Autodesk Fusion 360 part; units mm, degrees
(part 2 of 2)
sketch "20 mm Pickup Opening with Full-Height 45 Degree Bevel Lower Sketch" plane through (0, 0, 2) normal (0, 0, 1) x (1, 0, 0)
  line L0 (111.19, -12) -> (111.19, 37.0643)
  line L1 (111.19, 37.0643) -> (111.2756, 38.3696)
  line L2 (111.2756, 38.3696) -> (111.5307, 39.6525)
  line L3 (111.5307, 39.6525) -> (111.9512, 40.8911)
  line L4 (111.9512, 40.8911) -> (112.5297, 42.0643)
  line L5 (112.5297, 42.0643) -> (113.2565, 43.1519)
  line L6 (113.2565, 43.1519) -> (114.1189, 44.1354)
  line L7 (114.1189, 44.1354) -> (115.1024, 44.9978)
  line L8 (115.1024, 44.9978) -> (116.19, 45.7246)
  line L9 (116.19, 45.7246) -> (117.3632, 46.3031)
  line L10 (117.3632, 46.3031) -> (118.6018, 46.7236)
  line L11 (118.6018, 46.7236) -> (119.8847, 46.9787)
  line L12 (119.8847, 46.9787) -> (121.19, 47.0643)
  line L13 (121.19, 47.0643) -> (122.4953, 46.9787)
  line L14 (122.4953, 46.9787) -> (123.7782, 46.7236)
  line L15 (123.7782, 46.7236) -> (125.0168, 46.3031)
  line L16 (125.0168, 46.3031) -> (126.19, 45.7246)
  line L17 (126.19, 45.7246) -> (127.2776, 44.9978)
  line L18 (127.2776, 44.9978) -> (128.2611, 44.1354)
  line L19 (128.2611, 44.1354) -> (129.1235, 43.1519)
  line L20 (129.1235, 43.1519) -> (129.8503, 42.0643)
  line L21 (129.8503, 42.0643) -> (130.4288, 40.8911)
  line L22 (130.4288, 40.8911) -> (130.8493, 39.6525)
  line L23 (130.8493, 39.6525) -> (131.1044, 38.3696)
  line L24 (131.1044, 38.3696) -> (131.19, 37.0643)
  line L25 (131.19, 37.0643) -> (131.19, -12)
  line L26 (131.19, -12) -> (131.1044, -13.3053)
  line L27 (131.1044, -13.3053) -> (130.8493, -14.5882)
  line L28 (130.8493, -14.5882) -> (130.4288, -15.8268)
  line L29 (130.4288, -15.8268) -> (129.8503, -17)
  line L30 (129.8503, -17) -> (129.1235, -18.0876)
  line L31 (129.1235, -18.0876) -> (128.2611, -19.0711)
  line L32 (128.2611, -19.0711) -> (127.2776, -19.9335)
  line L33 (127.2776, -19.9335) -> (126.19, -20.6603)
  line L34 (126.19, -20.6603) -> (125.0168, -21.2388)
  line L35 (125.0168, -21.2388) -> (123.7782, -21.6593)
  line L36 (123.7782, -21.6593) -> (122.4953, -21.9144)
  line L37 (122.4953, -21.9144) -> (121.19, -22)
  line L38 (121.19, -22) -> (119.8847, -21.9144)
  line L39 (119.8847, -21.9144) -> (118.6018, -21.6593)
  line L40 (118.6018, -21.6593) -> (117.3632, -21.2388)
  line L41 (117.3632, -21.2388) -> (116.19, -20.6603)
  line L42 (116.19, -20.6603) -> (115.1024, -19.9335)
  line L43 (115.1024, -19.9335) -> (114.1189, -19.0711)
  line L44 (114.1189, -19.0711) -> (113.2565, -18.0876)
  line L45 (113.2565, -18.0876) -> (112.5297, -17)
  line L46 (112.5297, -17) -> (111.9512, -15.8268)
  line L47 (111.9512, -15.8268) -> (111.5307, -14.5882)
  line L48 (111.5307, -14.5882) -> (111.2756, -13.3053)
  line L49 (111.2756, -13.3053) -> (111.19, -12)
sketch "20 mm Pickup Opening with Full-Height 45 Degree Bevel Upper Sketch" plane through (0, 0, 10.2) normal (0, 0, 1) x (1, 0, 0)
  line L0 (102.99, -20.2) -> (102.99, 45.2643)
  line L1 (102.99, 45.2643) -> (103.1457, 47.6399)
  line L2 (103.1457, 47.6399) -> (103.6101, 49.9748)
  line L3 (103.6101, 49.9748) -> (104.3754, 52.2291)
  line L4 (104.3754, 52.2291) -> (105.4283, 54.3643)
  line L5 (105.4283, 54.3643) -> (106.751, 56.3438)
  line L6 (106.751, 56.3438) -> (108.3207, 58.1336)
  line L7 (108.3207, 58.1336) -> (110.1105, 59.7033)
  line L8 (110.1105, 59.7033) -> (112.09, 61.026)
  line L9 (112.09, 61.026) -> (114.2252, 62.0789)
  line L10 (114.2252, 62.0789) -> (116.4795, 62.8441)
  line L11 (116.4795, 62.8441) -> (118.8144, 63.3086)
  line L12 (118.8144, 63.3086) -> (121.19, 63.4643)
  line L13 (121.19, 63.4643) -> (123.5656, 63.3086)
  line L14 (123.5656, 63.3086) -> (125.9005, 62.8441)
  line L15 (125.9005, 62.8441) -> (128.1548, 62.0789)
  line L16 (128.1548, 62.0789) -> (130.29, 61.026)
  line L17 (130.29, 61.026) -> (132.2695, 59.7033)
  line L18 (132.2695, 59.7033) -> (134.0593, 58.1336)
  line L19 (134.0593, 58.1336) -> (135.629, 56.3438)
  line L20 (135.629, 56.3438) -> (136.9517, 54.3643)
  line L21 (136.9517, 54.3643) -> (138.0046, 52.2291)
  line L22 (138.0046, 52.2291) -> (138.7699, 49.9748)
  line L23 (138.7699, 49.9748) -> (139.2343, 47.6399)
  line L24 (139.2343, 47.6399) -> (139.39, 45.2643)
  line L25 (139.39, 45.2643) -> (139.39, -20.2)
  line L26 (139.39, -20.2) -> (139.2343, -22.5756)
  line L27 (139.2343, -22.5756) -> (138.7699, -24.9105)
  line L28 (138.7699, -24.9105) -> (138.0046, -27.1648)
  line L29 (138.0046, -27.1648) -> (136.9517, -29.3)
  line L30 (136.9517, -29.3) -> (135.629, -31.2795)
  line L31 (135.629, -31.2795) -> (134.0593, -33.0693)
  line L32 (134.0593, -33.0693) -> (132.2695, -34.639)
  line L33 (132.2695, -34.639) -> (130.29, -35.9617)
  line L34 (130.29, -35.9617) -> (128.1548, -37.0146)
  line L35 (128.1548, -37.0146) -> (125.9005, -37.7799)
  line L36 (125.9005, -37.7799) -> (123.5656, -38.2443)
  line L37 (123.5656, -38.2443) -> (121.19, -38.4)
  line L38 (121.19, -38.4) -> (118.8144, -38.2443)
  line L39 (118.8144, -38.2443) -> (116.4795, -37.7799)
  line L40 (116.4795, -37.7799) -> (114.2252, -37.0146)
  line L41 (114.2252, -37.0146) -> (112.09, -35.9617)
  line L42 (112.09, -35.9617) -> (110.1105, -34.639)
  line L43 (110.1105, -34.639) -> (108.3207, -33.0693)
  line L44 (108.3207, -33.0693) -> (106.751, -31.2795)
  line L45 (106.751, -31.2795) -> (105.4283, -29.3)
  line L46 (105.4283, -29.3) -> (104.3754, -27.1648)
  line L47 (104.3754, -27.1648) -> (103.6101, -24.9105)
  line L48 (103.6101, -24.9105) -> (103.1457, -22.5756)
  line L49 (103.1457, -22.5756) -> (102.99, -20.2)
loft "20 mm Pickup Opening with Full-Height 45 Degree Bevel" cut profiles "20 mm Pickup Opening with Full-Height 45 Degree Bevel Lower Sketch", "20 mm Pickup Opening with Full-Height 45 Degree Bevel Upper Sketch" section 1 section 2
equation "tableWidth = 200.0 mm" comment "Assumed table width"
equation "insideStopSpan = 250.0 mm" comment "Side-stop inside span"
equation "baseThickness = 2.0 mm" comment "Wafer support base"
equation "sidewallHeight = 1.5 mm" comment "Wall above support base"
equation "tableLipDrop = 5.0 mm" comment "Table contact below base"
equation "strutWidth = 8.0 mm" comment "PLA top-rib width"
equation "strutHeight = 8.0 mm" comment "PLA top-rib height above base"
equation "ribEndHeight = 1.5 mm" comment "Rib height where it meets nest"
equation "pickupChamfer = 8.0 mm" comment "45 degree pickup-slot bevel"
equation "pickupGapWidth = 20.0 mm" comment "Primary-flat pickup opening"
